Autodesk Fusion 360 part; units mm, degrees
note: some values were not read from the file. Chosen so that the rebuilt part matches the saved one: which face or edge a step refers to; the layout of a text; which pieces of a blend or face edit are solid.
(part 2 of 2)
  spline S203 degree 3 poles (-16.4478, 16.3049) (-16.4086, 16.3418) (-16.3228, 16.4228) (-16.2792, 16.5328) (-16.2555, 16.5925) knots 0 0 0 0 0.015968 0.034972 0.034972 0.034972 0.034972
  line L149 (-16.2555, 16.5925) -> (-15.9332, 16.5528)
  spline S204 degree 3 poles (-15.9332, 16.5528) (-15.9628, 16.4648) (-16.0201, 16.2947) (-16.1519, 16.1731) (-16.2155, 16.1143) knots 0 0 0 0 0.027335 0.052898 0.052898 0.052898 0.052898
  spline S205 degree 3 poles (-16.2155, 16.1143) (-16.2918, 16.0689) (-16.4537, 15.9724) (-16.6424, 15.9631) (-16.7422, 15.9583) knots 0 0 0 0 0.026229 0.055682 0.055682 0.055682 0.055682
  spline S206 degree 3 poles (-16.7422, 15.9583) (-16.8678, 15.9666) (-17.108, 15.9824) (-17.2938, 16.1343) (-17.3825, 16.2067) knots 0 0 0 0 0.03672 0.070219 0.070219 0.070219 0.070219
  spline S207 degree 3 poles (-17.3825, 16.2067) (-17.4514, 16.3028) (-17.6002, 16.5103) (-17.6125, 16.7665) (-17.6192, 16.904) knots 0 0 0 0 0.034736 0.075044 0.075044 0.075044 0.075044
  spline S208 degree 3 poles (-17.6192, 16.904) (-17.6127, 17.0462) (-17.6007, 17.31) (-17.4498, 17.5255) (-17.3802, 17.6249) knots 0 0 0 0 0.041667 0.077342 0.077342 0.077342 0.077342
  spline S209 degree 3 poles (-17.3802, 17.6249) (-17.2932, 17.6997) (-17.1149, 17.8529) (-16.8802, 17.8718) (-16.76, 17.8815) knots 0 0 0 0 0.033526 0.068681 0.068681 0.068681 0.068681
  spline S210 degree 3 poles (-16.76, 17.8815) (-16.6435, 17.8719) (-16.4151, 17.8532) (-16.2419, 17.7036) (-16.157, 17.6304) knots 0 0 0 0 0.034109 0.066844 0.066844 0.066844 0.066844
  spline S211 degree 3 poles (-16.157, 17.6304) (-16.0889, 17.533) (-15.9411, 17.3216) (-15.9293, 17.063) (-15.9229, 16.9235) knots 0 0 0 0 0.034955 0.075832 0.075832 0.075832 0.075832
  spline S212 degree 3 poles (-15.9229, 16.9235) (-15.923, 16.912) (-15.9233, 16.8843) (-15.9242, 16.8565) (-15.9246, 16.8404) knots 0 0 0 0 0.003465 0.008319 0.008319 0.008319 0.008319
  line L150 (-15.9246, 16.8404) -> (-17.2969, 16.84)
  spline S213 degree 3 poles (-17.2969, 16.84) (-17.2878, 16.7476) (-17.2712, 16.5772) (-17.1711, 16.439) (-17.1252, 16.3757) knots 0 0 0 0 0.027261 0.050297 0.050297 0.050297 0.050297
  spline S214 degree 3 poles (-17.1252, 16.3757) (-17.0703, 16.3287) (-16.9594, 16.2339) (-16.8139, 16.2211) (-16.7405, 16.2147) knots 0 0 0 0 0.021124 0.042643 0.042643 0.042643 0.042643
  line L151 (-19.2842, -19.9234) -> (18.7515, -19.9234) construction
  line L152 (18.7515, -19.9234) -> (18.7515, -15.0225) construction
  line L153 (18.7515, -15.0225) -> (-19.2842, -15.0225) construction
  line L154 (-19.2842, -15.0225) -> (-19.2842, -19.9234) construction
  dimension "d40" = 2.54
  text T0 "https://AtlasRV.Solutions" font "Arial" height 2.54 align left top in box 38.0357 x 4.901 at (-19.2842, -19.9234) x (1, 0) y (0, 1) spacing 1 kerned
extrude "Extrude8" cut sketch "Sketch8" against normal blind 0.762 text T0
sketch "Sketch9" plane through (0, 0, 2.54) normal (0, 0, 1) x (1, 0, 0)
  circle A0 centre (-12.8169, 12.7) radius 6.731
  circle A1 centre (0, 0) radius 5.08
  circle A2 centre (12.4408, 12.7033) radius 6.731
  line L0 (21.336, 21.336) -> (-21.336, 21.336)
  line L1 (-21.336, 21.336) -> (-21.336, -21.336)
  line L2 (-21.336, -21.336) -> (21.336, -21.336)
  line L3 (21.336, -21.336) -> (21.336, 21.336)
  circle A3 centre (-0.1065, 7.5645) radius 2.54
  circle A4 centre (-0.1065, -7.6711) radius 2.54
  dimension "d48" = 5.08
  dimension "d49" = 5.08
  measures "d48" diameter of A3
  measures "d49" diameter of A4
extrude "Extrude9" add sketch "Sketch9" along normal blind 12.7 contours A1 A3 | A1 A3 | A4 picked at (-0.31, 5.0525) picked at (-0.0008, 8.4243)
sketch "Sketch10" plane through (0, 0, 2.54) normal (0, 0, 1) x (1, 0, 0)
  circle A0 centre (-0.1065, -7.6711) radius 2.54
  circle A1 centre (-12.8169, 12.7) radius 6.731
  circle A2 centre (12.4408, 12.7033) radius 6.731
  line L0 (21.336, 21.336) -> (-21.336, 21.336)
  line L1 (-21.336, 21.336) -> (-21.336, -21.336)
  line L2 (-21.336, -21.336) -> (21.336, -21.336)
  line L3 (21.336, -21.336) -> (21.336, 21.336)
  line L4 (-21.336, -21.415) -> (21.5216, -21.415) construction
  line L5 (21.5216, -21.415) -> (21.5216, -9.6954) construction
  line L6 (21.5216, -9.6954) -> (-21.336, -9.6954) construction
  line L7 (-21.336, -9.6954) -> (-21.336, -21.415) construction
  arc A3 (0.358, 5.0674) -> (-0.5006, 5.0553) centre (-0.1065, 7.5645) ccw
  arc A4 (-0.5006, 5.0553) -> (0.358, 5.0674) centre (0, 0) ccw
  dimension "d52" = 2.54
  text T0 "Vekooto Antenna Bracket\nv1.3 PETG\nhttps://AtlasRV.solutions" font "Arial" height 2.54 align centre top in box 42.8576 x 11.7197 at (-21.336, -21.415) x (1, 0) y (0, 1) spacing 1 kerned
  constraint coincident L1
extrude "Extrude10" add sketch "Sketch10" along normal blind 0.762 text T0
pattern_circular "C-Pattern1" [suppressed]
equation "plateWidth = 0.88 * 2 in"
equation "holeDiameter = 0.4 in"
equation "plateThickness = 0.1 in"
equation "d4 = plateWidth"
equation "d5 = plateWidth"
equation "d6 = plateThickness"
equation "d8 = holeDiameter"
equation "d9 = -plateThickness"
equation "postDiameter = 0.35 in"
equation "postHeight = 2 in"
equation "d13 = postDiameter"
equation "d14 = postHeight"
equation "d18 = postDiameter"
equation "d19 = postHeight"
equation "postCoreDiameter = 0.2 in"
equation "d22 = postCoreDiameter"
equation "d23 = postCoreDiameter"
equation "d24 = -postHeight"
equation "d26 = -postHeight"
equation "d37 = 'Vekooto Antenna Bracket v.1.1'"
equation "d41 = 'https://AtlasRV.Solutions'"
equation "antennaKnobDiameter = 0.5 in"
equation "antennaKnobOffset = 0.5 in"
equation "standoffStudDiameter = 0.2 in"
equation "d48 = standoffStudDiameter"
equation "d49 = standoffStudDiameter"
equation "d50 = antennaKnobOffset"
equation "d53 = 'Vekooto Antenna Bracket v1.3 PETG https://AtlasRV.solutions'"
